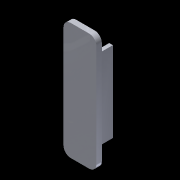
# Autodesk Inventor part: Belt Aligner MagLock
Saved by Autodesk Inventor 2014 SP1 (Build 180222100, 222)
## iProperties
Created: 2013-12-03
Part Number: Belt Aligner MagLock
Material: Polyethylene, High Density
Document SubType Name: Modeling
Designer: Rauhul Varma
Mass: 17.8594 g
Surface Area: 108.509 cm^2
Volume: 18.7599 cm^3
Density: 0.952 g/cm^3
Appearance: Ice White
Author: Rauhul Varma
Autodesk Inventor part; units mm, degrees
ref_plane "YZ Plane" through (0, 0, 0) normal (1, 0, 0) x (0, 1, 0)
ref_plane "XZ Plane" through (0, 0, 0) normal (0, 1, 0) x (-1, 0, 0)
ref_plane "XY Plane" through (0, 0, 0) normal (0, 0, 1) x (1, 0, 0)
sketch "Sketch1" plane through (0, 0, 0) normal (0, 0, 1) x (1, 0, 0)
  line L0 (0, 0) -> (50.8, 0) construction
  line L1 (50.8, 0) -> (50.8, 127) construction
  line L2 (50.8, 127) -> (0, 127) construction
  line L3 (0, 127) -> (0, 0) construction
  line L4 (0, 63.5) -> (50.8, 63.5) construction
  line L5 (25.4, 127) -> (25.4, 0) construction
  line L6 (6.7469, 46) -> (44.0531, 46) construction
  line L7 (44.0531, 46) -> (44.0531, 81) construction
  line L8 (44.0531, 81) -> (6.7469, 81) construction
  line L9 (6.7469, 81) -> (6.7469, 46) construction
  line L10 (41.6177, 127) -> (41.6177, 0) construction
  line L11 (26.6177, 127) -> (26.6177, 0) construction
  line L12 (45.2437, 28.575) -> (45.2437, 98.425)
  line L13 (45.2437, 98.425) -> (22.9917, 98.425)
  line L14 (22.9917, 98.425) -> (22.9917, 28.575)
  line L15 (22.9917, 28.575) -> (45.2437, 28.575)
  line L16 (42.0688, 28.575) -> (42.0688, 98.425)
  line L17 (26.1667, 28.575) -> (26.1667, 98.425)
  line L18 (24.5927, 22.225) -> (43.6427, 22.225)
  line L19 (43.6427, 22.225) -> (43.6427, 15.875)
  line L20 (43.6427, 15.875) -> (24.5927, 15.875)
  line L21 (24.5927, 15.875) -> (24.5927, 22.225)
  line L22 (34.1177, 0) -> (34.1177, 127) construction
  line L23 (43.6427, 111.125) -> (24.5927, 111.125)
  line L24 (24.5927, 111.125) -> (24.5927, 104.775)
  line L25 (24.5927, 104.775) -> (43.6427, 104.775)
  line L26 (43.6427, 104.775) -> (43.6427, 111.125)
  line L27 (19.8302, 12.7) -> (48.4052, 12.7)
  line L28 (48.4052, 12.7) -> (48.4052, 114.3)
  line L29 (48.4052, 114.3) -> (19.8302, 114.3)
  line L30 (19.8302, 114.3) -> (19.8302, 12.7)
  dimension "d0" = 50.8
  dimension "d1" = 127
  dimension "d2" = 35
  dimension "d3" = 37.3062
  dimension "d4" = 15
  dimension "d5" = 2.4354
  dimension "d6" = 5.5563
  dimension "d7" = 3.175
  dimension "d8" = 0.451
  dimension "d9" = 0.451
  dimension "d10" = 3.175
  dimension "d11" = 69.85
  dimension "d12" = 19.05
  dimension "d13" = 6.35
  dimension "d14" = 6.35
  dimension "d15" = 6.35
  dimension "d16" = 19.05
  dimension "d17" = 6.35
  dimension "d18" = 3.175
  dimension "d21" = 3.175
  dimension "d30" = 28.575
  dimension "d32" = 3.1615
  dimension "d33" = 3.1615
  constraints: 62 end point, 13 parallel, 11 perpendicular, 10 point on line, 5 horizontal, 4 midpoint, 7 other
  measures "d0" distance of L2.end L1.end
  measures "d1" distance of L1.end L0.end
  measures "d2" distance between parallel lines of L6 L8
  measures "d3" distance between parallel lines of L7 L9
  measures "d4" distance between parallel lines of L10 L11
  measures "d5" distance between parallel lines of L7 L10
  measures "d6" distance between parallel lines of L1 L12
  measures "d7" distance between parallel lines of L12 L16
  measures "d8" distance between parallel lines of L16 L10
  measures "d9" distance between parallel lines of L17 L11
  measures "d10" distance between parallel lines of L14 L17
  measures "d11" distance between parallel lines of L15 L13
  measures "d12" distance between parallel lines of L19 L21
  measures "d13" distance between parallel lines of L20 L18
  measures "d14" distance between parallel lines of L15 L18
  measures "d15" distance between parallel lines of L25 L23
  measures "d16" distance between parallel lines of L26 L24
  measures "d17" distance between parallel lines of L13 L25
  measures "d18" distance between parallel lines of L27 L20
  measures "d21" distance between parallel lines of L29 L23
  measures "d30" distance between parallel lines of L30 L28
  measures "d32" distance between parallel lines of L30 L14
  measures "d33" distance between parallel lines of L28 L12
extrude "Main Cover Profile" add sketch "Sketch1" along normal blind 4.7625 contours L15 L16 L13 L12 | L15 L17 L13 L16 | L15 L14 L13 L17 | L18 L19 L20 L21 | L26 L25 L24 L23 | L30 L29 L28 L27
extrude "Magnet Pockets" cut sketch "Sketch1" along normal blind 2.3813 contours L18 L19 L20 L21 | L26 L25 L24 L23
extrude "Belt Aligning Tabs" add sketch "Sketch1" against normal blind 12.7 contours L15 L16 L13 L12 | L15 L14 L13 L17
fillet "Fillet1" radius 3.175 8 edges at (43.6427, 22.225, 1.1906) (43.6427, 15.875, 1.1906) (24.5927, 15.875, 1.1906) (24.5927, 22.225, 1.1906) (43.6427, 104.775, 1.1906) (43.6427, 111.125, 1.1906) (24.5927, 104.775, 1.1906) (24.5927, 111.125, 1.1906)
fillet "Fillet2" radius 6.35 4 edges at (48.4052, 114.3, 2.3813) (48.4052, 12.7, 2.3813) (19.8302, 12.7, 2.3813) (19.8302, 114.3, 2.3813)
equation "\"d5\" = -0.666667 * d4 + 0.333333 * d3"
equation "\"d9\" = d8"
equation "\"d10\" = d7"
equation "\"d12\" = d16"
equation "\"d13\" = d15"
body "Solid1"
